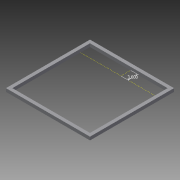
# Autodesk Inventor part: Frame Outline
Saved by Autodesk Inventor 2015 (Build 190159000, 159)
## iProperties
Created: 2015-01-08
Part Number: Frame Outline
Material: Generic
Document SubType Name: Modeling
Designer: jhirshland1
Density: 1 g/cm^3
Appearance: Default
Author: jhirshland1
Autodesk Inventor part; units mm, degrees
ref_plane "YZ Plane" through (0, 0, 0) normal (1, 0, 0) x (0, 1, 0)
ref_plane "XZ Plane" through (0, 0, 0) normal (0, 1, 0) x (-1, 0, 0)
ref_plane "XY Plane" through (0, 0, 0) normal (0, 0, 1) x (1, 0, 0)
sketch "Sketch1" plane through (0, 0, 0) normal (0, 1, 0) x (-1, 0, 0)
  line L0 (8.7651, 9.9871) -> (-651.6349, 9.9871)
  line L1 (-651.6349, 9.9871) -> (-651.6349, -650.4129)
  line L2 (-651.6349, -650.4129) -> (8.7651, -650.4129)
  line L3 (8.7651, -650.4129) -> (8.7651, 9.9871)
  line L4 (-16.6349, -15.4129) -> (-626.2349, -15.4129)
  line L5 (-626.2349, -15.4129) -> (-626.2349, -625.0129)
  line L6 (-626.2349, -625.0129) -> (-16.6349, -625.0129)
  line L7 (-16.6349, -625.0129) -> (-16.6349, -15.4129)
  point P0 (0, 0)
  dimension "d0" = 660.4
  dimension "d1" = 660.4
  dimension "d2" = 25.4
  constraints: 16 end point, 4 parallel, 2 perpendicular, 1 horizontal, 3 other
  measures "d0" distance of L2.end L1.end
  measures "d1" distance of L1.end L0.end
  measures "d2" distance between parallel lines of L3 L7
sketch "Sketch2" plane through (0, 0, 0) normal (0, 1, 0) x (-1, 0, 0)
  line L0 (-333.5663, -626.2819) -> (-333.5663, -550.0819) construction
  line L1 (-625.3108, -550.0819) -> (-18.6287, -550.0819) construction
  point P0 (0, 0)
  dimension "d3" = 76.2
  constraints: 4 end point, 1 horizontal, 1 vertical
  measures "d3" distance of L0.start L0.end
extrude "Extrusion1" add sketch "Sketch1" along normal blind 25.4
body "Solid1"
